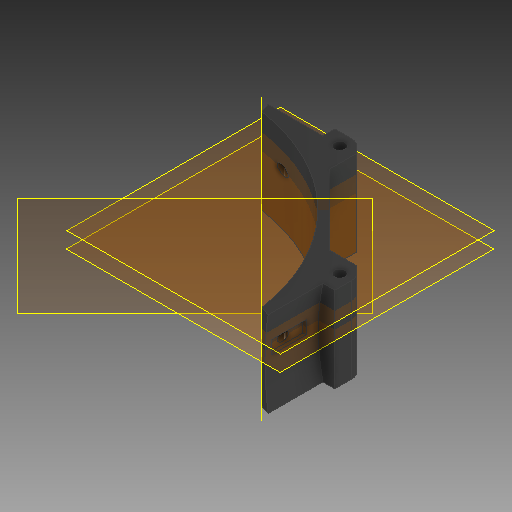
# Autodesk Inventor part: kicker_cetch
Saved by Autodesk Inventor 2020 (Build 240168000, 168)
## iProperties
Created: 2024-09-29
Part Number: kicker_cetch
Material: Типовые
Document SubType Name: Modeling
Designer: Ivan
Density: 1 g/cm^3
Appearance: Черный — литой
Author: Ivan
Autodesk Inventor part; units mm, degrees
ref_plane "YZ Plane" through (0, 0, 0) normal (1, 0, 0) x (0, 1, 0)
ref_plane "XZ Plane" through (0, 0, 0) normal (0, 1, 0) x (-1, 0, 0)
ref_plane "XY Plane" through (0, 0, 0) normal (0, 0, 1) x (1, 0, 0)
sketch "Эскиз1" plane through (0, 0, 0) normal (0, 1, 0) x (-1, 0, 0)
  circle A0 centre (-44.87, 82.9015) radius 1.5
  line L0 (-31, 99.2724) -> (-31, 78.7724)
  line L1 (-31, 78.7724) -> (31, 78.7724)
  circle A1 centre (-42.22, 16) radius 1.5
  circle A2 centre (-16, 42.22) radius 1.5
  circle A3 centre (16, 42.22) radius 1.5
  circle A4 centre (31, 72.43) radius 1.5
  circle A5 centre (16, 72.43) radius 1.5
  circle A6 centre (-16, 72.43) radius 1.5
  arc A7 (-31, 99.2724) -> (-99.2724, 31) centre (0, 0) ccw
  circle A8 centre (-74.5664, 57.67) radius 1.5
  circle A9 centre (-82.9015, 44.87) radius 1.5
  circle A10 centre (-72.43, -16) radius 1.5
  circle A11 centre (-72.43, 16) radius 1.5
  line L2 (-78.7724, 31) -> (-78.7724, -31)
  line L3 (-99.2724, 31) -> (-78.7724, 31)
  line L4 (31, 78.7724) -> (31, 99.2724)
  arc A12 (34.57, 98.0863) -> (98.0863, 34.57) centre (109.0212, 109.0212) ccw
  circle A13 centre (72.43, 31) radius 1.5
  line L5 (99.2724, 31) -> (78.7724, 31)
  circle A14 centre (72.43, 16) radius 1.5
  arc A15 (34.57, 98.0863) -> (31, 99.2724) centre (0, 0) ccw
  arc A16 (99.2724, 31) -> (98.0863, 34.57) centre (0, 0) ccw
  arc A17 (98.0863, 34.57) -> (34.57, 98.0863) centre (0, 0) ccw
  circle A18 centre (42.22, 16) radius 1.5
  circle A19 centre (82.9015, -44.87) radius 1.5
  line L6 (78.7724, -31) -> (99.2724, -31)
  arc A20 (31, -99.2724) -> (99.2724, -31) centre (0, 0) ccw
  circle A21 centre (16, -72.43) radius 1.5
  line L7 (31, -78.7724) -> (31, -99.2724)
  circle A22 centre (44.87, -82.9015) radius 1.5
  circle A23 centre (57.67, -74.5664) radius 1.5
  circle A24 centre (-57.67, 74.5664) radius 1.5
  circle A25 centre (-42.22, -16) radius 1.5
  circle A26 centre (42.22, -16) radius 1.5
  circle A27 centre (-72.43, -31) radius 1.5
  line L8 (-73.5391, 73.5391) -> (73.5391, -73.5391) construction
  line L9 (78.7724, 31) -> (78.7724, -31)
  circle A28 centre (72.43, -16) radius 1.5
  circle A29 centre (-16, -42.22) radius 1.5
  circle A30 centre (16, -42.22) radius 1.5
  circle A31 centre (74.5664, -57.67) radius 1.5
  line L10 (-31, -78.7724) -> (31, -78.7724)
  circle A32 centre (-16, -72.43) radius 1.5
  circle A33 centre (-31, -72.43) radius 1.5
  line L11 (-31, -99.2724) -> (-31, -78.7724)
  arc A34 (-34.57, -98.0863) -> (-31, -99.2724) centre (0, 0) ccw
  line L12 (-78.7724, -31) -> (-99.2724, -31)
  arc A35 (-99.2724, -31) -> (-98.0863, -34.57) centre (0, 0) ccw
  arc A36 (-98.0863, -34.57) -> (-34.57, -98.0863) centre (0, 0) ccw
  arc A37 (-34.57, -98.0863) -> (-98.0863, -34.57) centre (-109.0212, -109.0212) ccw
  constraints: 38 centre point, 26 end point, 23 point on circle, 5 coincident, 1 horizontal, 1 perpendicular, 1 symmetric about line, 2 other
sketch "Эскиз2" plane through (0, 0, 0) normal (0, 1, 0) x (-1, 0, 0)
  arc A0 (34.57, 98.0863) -> (98.0863, 34.57) centre (109.0212, 109.0212) ccw projected
  arc A1 (99.2724, 31) -> (98.0863, 34.57) centre (0, 0) ccw projected
  arc A2 (34.57, 98.0863) -> (31, 99.2724) centre (0, 0) ccw projected
  line L0 (31, 78.7724) -> (31, 99.2724) projected
  circle A3 centre (31, 72.43) radius 1.5 projected
  circle A4 centre (72.43, 31) radius 1.5 projected
  circle A5 centre (31, 72.43) radius 4.5
  circle A6 centre (72.43, 31) radius 4.5
  line L1 (27.818, 69.248) -> (69.248, 27.818)
  line L2 (26.5, 78.7724) -> (26.5, 72.43)
  line L3 (78.7724, 31) -> (78.7724, -31) projected
  line L4 (78.7724, 26.5) -> (72.43, 26.5)
  line L5 (99.2724, 31) -> (78.7724, 31) projected
  line L6 (26.5, 78.7724) -> (31, 78.7724)
  dimension "d0" = 9
  dimension "d1" = 9
  constraints: 8 end point, 4 point on circle, 4 tangent, 2 centre point, 2 coincident, 2 horizontal, 1 point on line, 1 vertical
  measures "d0" diameter of A5
  measures "d1" diameter of A6
extrude "Выдавливание1" add sketch "Эскиз2" along normal blind 32
ref_plane "РабПлоскость1" through (0, 25.3, 0) normal (0, 1, 0) x (1, 0, 0)
sketch "Эскиз3" plane through (0, 25.3, 0) normal (0, 1, 0) x (1, 0, 0)
  circle A0 centre (-72.43, -31) radius 1.5 projected
  circle A1 centre (-31, -72.43) radius 1.5 projected
  point P0 (0, 0)
extrude "Выдавливание2" add sketch "Эскиз3" against normal blind 20.6
sketch "Эскиз4" plane through (-31, 0, 78.7724) normal (0, 0, 1) x (1, 0, 0)
  line L0 (0, 1) -> (0, 32)
  line L1 (0, 32) -> (-3.57, 32) projected
  line L2 (0, 0) -> (0, 32) projected
  arc A0 (0, 32) -> (0, 0) centre (72.5929, 16) ccw
  point P0 (31, 0)
  constraints: 2 end point, 2 point on circle, 1 centre point, 1 vertical
extrude "Выдавливание3" cut sketch "Эскиз4" along normal through all
ref_plane "РабПлоскость2" through (-48.533, 0, 48.533) normal (0.7071068, 0, 0.7071068) x (0, 1, 0)
mirror "Зеркальное отражение1" about plane through (-48.533, 0, 48.533) normal (0.7071068, 0, 0.7071068) of "Выдавливание3"
ref_plane "РабПлоскость3" through (-98.0863, 32, 34.57) normal (0.7071068, 0, -0.7071068) x (0.7071068, 0, 0.7071068)
sketch "Эскиз6" plane through (-98.0863, 32, 34.57) normal (0.7071068, 0, -0.7071068) x (0.7071068, 0, 0.7071068)
  line L0 (0, -5.66) -> (89.8256, -5.66)
  line L1 (89.8256, -5.66) -> (89.8256, 35)
  line L2 (89.8256, 35) -> (0, 35)
  line L3 (0, 35) -> (0, -5.66)
  circle A0 centre (45.1056, 17) radius 2
  line L4 (89.8256, 32) -> (89.8256, 0) projected
  line L5 (89.8256, 32) -> (89.8256, 35)
  point P0 (44.9128, 32)
  dimension "d12" = 3
  constraints: 10 end point, 2 parallel, 1 centre point, 1 horizontal, 1 perpendicular, 1 vertical
  measures "d12" distance of L4.start L5.end
hole "Отверстие1" at (-66.1918, 15, 66.4645) direction (0.7071068, 0, -0.7071068) diameter 5.5 end through all
sketch "Эскиз7" plane through (0, 32, 0) normal (0, 1, 0) x (1, 0, 0)
  line L0 (-31, -78.7724) -> (-26.5, -78.7724) construction
  line L1 (-78.7724, -26.5) -> (-78.7724, -31) construction
  line L2 (-31, -78.7724) -> (-78.7724, -31) construction
  arc A0 (-34.57, -98.0863) -> (-98.0863, -34.57) centre (-109.0212, -109.0212) ccw construction
  line L3 (-40.6087, -66.7716) -> (-66.7716, -40.6087)
  line L4 (-66.7716, -40.6087) -> (-66.7716, -30.2944)
  line L5 (-66.7716, -40.6087) -> (-61.6145, -35.4515) construction
  line L6 (152.6297, 152.6297) -> (-152.6297, -152.6297) construction
  line L7 (-61.6145, -35.4515) -> (-66.7716, -30.2944) construction
  line L8 (-27.818, -69.248) -> (-69.248, -27.818) construction
  line L9 (-40.6087, -66.7716) -> (-30.2944, -66.7716)
  line L10 (-40.6087, -66.7716) -> (-35.4515, -61.6145) construction
  line L11 (-35.4515, -61.6145) -> (-30.2944, -66.7716) construction
  line L12 (-30.2944, -66.7716) -> (-66.7716, -30.2944)
  point P0 (0, 0)
  point P1 (-55.8115, -55.8115)
  point P2 (-53.6901, -53.6901)
  dimension "d20" = 3
  dimension "d21" = 37
  constraints: 18 end point, 3 point on line, 2 perpendicular, 2 symmetric about line, 1 midpoint, 1 parallel, 1 point on circle
  measures "d20" distance from line of L3 point (-55.811, -55.811)
  measures "d21" distance from line of L5 L3.start
extrude "Выдавливание4" cut sketch "Эскиз7" against normal through all
ref_plane "РабПлоскость4" through (0, 19.2, 0) normal (0, 1, 0) x (1, 0, 0)
sketch "Эскиз9" plane through (0, 32, 0) normal (0, 1, 0) x (1, 0, 0)
  arc A0 (-98.0863, -34.57) -> (-34.57, -98.0863) centre (0, 0) ccw projected
  arc A1 (-34.57, -98.0863) -> (-98.0863, -34.57) centre (-109.0212, -109.0212) ccw construction
  line L0 (-73.5391, -73.5391) -> (-55.8115, -55.8115)
  line L1 (-89.442, -36.363) -> (-31, -94.805)
  line L2 (-31, -99.2724) -> (-31, -78.7724) construction
  line L3 (-218.9579, 86.3016) -> (86.3016, -218.9579) projected
  line L4 (-32.7423, -78.7724) -> (-32.7423, -98.7114) projected
  line L5 (-25, -115) -> (25, -115) construction
  line L6 (25, -115) -> (25, -87) construction
  line L7 (25, -87) -> (-25, -87) construction
  line L8 (-25, -87) -> (-25, -115) construction
  line L9 (31, -78.7724) -> (-31, -78.7724) projected
  line L10 (0, -78.7724) -> (0, -128.7724) construction
  line L11 (-37, -86) -> (-32.6866, -81.6866)
  line L12 (-32.6866, -81.6866) -> (-24.2014, -90.1719)
  line L13 (-24.2014, -90.1719) -> (-28.5147, -94.4853)
  line L14 (-28.5147, -94.4853) -> (-37, -86)
  point P0 (-62.9025, -62.9025)
  point P1 (0, -87)
  dimension "d25" = 17.7276
  dimension "d26" = 7.0911
  dimension "d35" = 50
  dimension "d36" = 50
  dimension "d38" = 6.1
  dimension "d39" = 12
  constraints: 22 end point, 6 parallel, 4 point on line, 3 point on circle, 2 midpoint, 2 perpendicular, 1 horizontal, 1 vertical
  measures "d25" horizontal distance of L0.start L0.end
  measures "d26" horizontal distance of point (-62.903, -62.903) L0.end
  measures "d35" distance of L7.end L6.end
  measures "d36" distance of L10.start L10.end
  measures "d38" distance from line of L12 L11.start
  measures "d39" distance from line of L11 L13.end
sketch "Эскиз10" plane through (0, 19.2, 0) normal (0, 1, 0) x (1, 0, 0)
  line L0 (-34, -83.2724) -> (-34, -96.2724)
  line L1 (-34, -96.2724) -> (-31, -96.2724)
  line L2 (-31, -96.2724) -> (-31, -83.2724)
  line L3 (-31, -83.2724) -> (-34, -83.2724)
  line L4 (-31, -99.2724) -> (-31, -78.7724) projected
  arc A0 (-34.57, -98.0863) -> (-31, -99.2724) centre (0, 0) ccw projected
  point P0 (-31, -99.2724)
  dimension "d40" = 3
  dimension "d41" = 13
  dimension "d65" = 3
  constraints: 8 end point, 3 parallel, 1 coincident, 1 perpendicular
  measures "d40" distance from line of L2 L0.start
  measures "d41" distance from line of L1 L2.end
  measures "d65" distance of L1.end point (-31, -99.272)
extrude "Выдавливание6" cut sketch "Эскиз10" along normal mid plane 5.15
sketch "Эскиз11" plane through (-63.5, 13.425, 63.5) normal (0.7071068, 0, 0.7071068) x (0.7071068, 0, -0.7071068)
  circle A0 centre (1.6, 5.775) radius 1.5
  line L0 (15.3638, -13.425) -> (15.3638, 18.575) projected
  line L1 (6.8785, 3.2) -> (6.8785, 8.35) projected
  line L2 (6.8785, 5.775) -> (3.3286, 5.775)
  point P0 (89.8026, -13.425)
  dimension "d45" = 3
  dimension "d48" = 13.7638
  constraints: 2 end point, 1 centre point, 1 midpoint, 1 perpendicular, 1 point on line
  measures "d45" diameter of A0
  measures "d48" distance from line of L0 A0.centre
extrude "Выдавливание7" cut sketch "Эскиз11" along normal mid plane 100
sketch "Эскиз12" plane through (0, 32, 0) normal (0, 1, 0) x (1, 0, 0)
  circle A0 centre (-72.43, -31) radius 1.5 projected
  circle A1 centre (-31, -72.43) radius 1.5 projected
  point P0 (0, 0)
  constraints: 2 coincident
hole "Отверстие2" at (-72.43, 32, 31) at (-31, 32, 72.43) direction (0, -1, 0) diameter 4 depth 4.7
hole "Отверстие3" at (-31, 0, 72.43) at (-72.43, 0, 31) direction (0, 1, 0) diameter 4 depth 4.7
equation "\"d1\" = d0"
equation "\"d26\" = 0.4 * d25"
